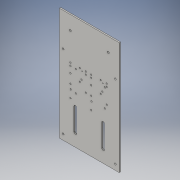
# Autodesk Inventor part: Part2
Saved by Autodesk Inventor 2016 (Build 200138000, 138)
## iProperties
Created: 2015-10-15
Part Number: Part2
Material: Generic
Document SubType Name: Modeling
Designer: hozhu
Density: 1 g/cm^3
Appearance: Default
Author: hozhu
Autodesk Inventor part; units mm, degrees
ref_plane "YZ Plane" through (0, 0, 0) normal (1, 0, 0) x (0, 1, 0)
ref_plane "XZ Plane" through (0, 0, 0) normal (0, 1, 0) x (-1, 0, 0)
ref_plane "XY Plane" through (0, 0, 0) normal (0, 0, 1) x (1, 0, 0)
sketch "Sketch1" plane through (0, 0, 0) normal (0, 0, 1) x (1, 0, 0)
  line L0 (-68.58, -128.7145) -> (68.58, -128.7145)
  line L1 (68.58, -128.7145) -> (68.58, 128.7145)
  line L2 (68.58, 128.7145) -> (-68.58, 128.7145)
  line L3 (-68.58, 128.7145) -> (-68.58, -128.7145)
  line L4 (-68.58, -128.7145) -> (68.58, 128.7145) construction
  line L5 (68.58, -128.7145) -> (-68.58, 128.7145) construction
  point P0 (0, 0)
  dimension "d0" = 137.16
  dimension "d1" = 257.429
  constraints: 12 end point, 2 midpoint, 2 parallel, 1 horizontal, 1 perpendicular
  measures "d0" distance of L1.end L2.end
  measures "d1" distance of L2.end L0.start
extrude "Extrusion1" add sketch "Sketch1" against normal blind 3.175
sketch "Sketch2" plane through (0, 0, 0) normal (0, 0, 1) x (1, 0, 0)
  circle A0 centre (-59.69, 52.5145) radius 2.0955
  line L0 (-68.58, 128.7145) -> (-68.58, -128.7145) projected
  line L1 (-68.58, 128.7145) -> (68.58, 128.7145) projected
  circle A1 centre (59.69, 52.5145) radius 2.0955
  line L2 (68.58, -128.7145) -> (68.58, 128.7145) projected
  circle A2 centre (-59.69, -116.0145) radius 2.0955
  circle A3 centre (59.69, -116.0145) radius 2.0955
  line L3 (-68.58, -128.7145) -> (68.58, -128.7145) projected
  point P0 (0, 0)
  dimension "d4" = 8.89
  dimension "d5" = 76.2
  dimension "d6" = 76.2
  dimension "d7" = 8.89
  dimension "d8" = 4.191
  dimension "d9" = 12.7
  dimension "d10" = 8.89
  dimension "d11" = 8.89
  dimension "d12" = 12.7
  dimension "d13" = 4.191
  dimension "d21" = 4.191
  dimension "d22" = 4.191
  constraints: 4 centre point
  measures "d4" distance from line of L0 A0.centre
  measures "d5" distance from line of L1 A0.centre
  measures "d6" distance from line of L1 A1.centre
  measures "d7" distance from line of A1.centre L2
  measures "d8" diameter of A1
  measures "d9" distance from line of L3 A2.centre
  measures "d10" distance from line of L0 A2.centre
  measures "d11" distance from line of L2 A3.centre
  measures "d12" distance from line of L3 A3.centre
  measures "d13" diameter of A0
  measures "d21" diameter of A2
  measures "d22" diameter of A3
hole "Hole1" at (-59.69, 52.5145, 0) at (59.69, 52.5145, 0) at (-59.69, -116.0145, 0) at (59.69, -116.0145, 0) direction (0, 0, -1) diameter 4.191 end through all
sketch "Sketch4" plane through (0, 0, 0) normal (0, 0, 1) x (1, 0, 0)
  line L0 (-35.179, -49.0855) -> (-35.179, -99.8855)
  line L1 (-28.321, -49.0855) -> (-28.321, -99.8855)
  line L2 (28.321, -49.0855) -> (28.321, -99.8855)
  line L3 (35.179, -49.0855) -> (35.179, -99.8855)
  line L4 (-68.58, 128.7145) -> (-68.58, -128.7145) projected
  line L5 (68.58, -128.7145) -> (68.58, 128.7145) projected
  line L6 (-68.58, -128.7145) -> (68.58, -128.7145) projected
  arc A0 (-28.321, -49.0855) -> (-35.179, -49.0855) centre (-31.75, -49.0855) ccw
  arc A1 (-35.179, -99.8855) -> (-28.321, -99.8855) centre (-31.75, -99.8855) ccw
  arc A2 (35.179, -49.0855) -> (28.321, -49.0855) centre (31.75, -49.0855) ccw
  arc A3 (28.321, -99.8855) -> (35.179, -99.8855) centre (31.75, -99.8855) ccw
  point P0 (0, 0)
  dimension "d23" = 6.858
  dimension "d24" = 6.858
  dimension "d25" = 33.401
  dimension "d26" = 50.8
  dimension "d27" = 33.401
  dimension "d28" = 28.829
  dimension "d29" = 28.829
  dimension "d30" = 28.829
  dimension "d31" = 28.829
  dimension "d32" = 50.8
  dimension "d33" = 50.8
  dimension "d34" = 50.8
  constraints: 8 end point, 8 point on circle, 4 centre point, 4 tangent, 4 vertical
  measures "d23" distance of L1.end L0.end
  measures "d24" distance between parallel lines of L3 L2
  measures "d25" distance between parallel lines of L4 L0
  measures "d26" distance of L3.start L3.end
  measures "d27" distance between parallel lines of L5 L3
  measures "d28" distance from line of L6 L0.end
  measures "d29" distance from line of L6 L1.end
  measures "d30" distance from line of L6 L2.end
  measures "d31" distance from line of L6 L3.end
  measures "d32" distance of L0.start L0.end
  measures "d33" distance of L1.start L1.end
  measures "d34" distance of L2.start L2.end
extrude "Extrusion2" cut sketch "Sketch4" against normal blind 3.175
sketch "Sketch5" plane through (0, 0, 0) normal (0, 0, 1) x (1, 0, 0)
  line L0 (-68.58, 128.7145) -> (68.58, 128.7145) projected
  line L1 (68.58, 128.7145) -> (68.58, -128.7145) projected
  point P0 (0, 0)
  point P1 (-43.3324, 96.9645)
  point P2 (43.3324, 96.9645)
  dimension "d37" = 31.75
  dimension "d38" = 86.6648
  dimension "d39" = 31.75
  dimension "d40" = 25.2476
  measures "d37" distance from line of L0 point (-43.332, 96.964)
  measures "d38" distance of point (-43.332, 96.964) point (43.332, 96.964)
  measures "d39" distance from line of L0 point (43.332, 96.964)
  measures "d40" distance from line of L1 point (43.332, 96.964)
hole "Hole2" at (-43.3324, 96.9645, 0) at (43.3324, 96.9645, 0) direction (0, 0, -1) diameter 4.4704 end through all
sketch "battery_buzzer" plane through (0, 0, 0) normal (0, 0, 1) x (1, 0, 0)
  line L0 (-50.8, 39.8145) -> (50.8, 39.8145)
  line L1 (50.8, 39.8145) -> (50.8, -36.3855)
  line L2 (50.8, -36.3855) -> (-50.8, -36.3855)
  line L3 (-50.8, -36.3855) -> (-50.8, 39.8145)
  line L4 (68.58, -128.7145) -> (68.58, 128.7145) projected
  line L5 (68.58, 128.7145) -> (-68.58, 128.7145) projected
  line L6 (-68.58, 128.7145) -> (-68.58, -128.7145) projected
  line L7 (-46.99, 37.2745) -> (-13.97, 37.2745)
  line L8 (-13.97, 37.2745) -> (-13.97, 9.3345)
  line L9 (-13.97, 9.3345) -> (-46.99, 9.3345)
  line L10 (-46.99, 9.3345) -> (-46.99, 37.2745)
  circle A0 centre (-43.18, 33.4645) radius 1.651
  circle A1 centre (-43.18, 12.5095) radius 1.651
  circle A2 centre (-17.78, 12.5095) radius 1.651
  line L11 (0.635, 37.2745) -> (33.655, 37.2745)
  line L12 (33.655, 37.2745) -> (33.655, 9.3345)
  line L13 (33.655, 9.3345) -> (0.635, 9.3345)
  line L14 (0.635, 9.3345) -> (0.635, 37.2745)
  circle A3 centre (4.445, 33.4645) radius 1.651
  circle A4 centre (4.445, 12.5095) radius 1.651
  circle A5 centre (29.845, 12.5095) radius 1.651
  point P0 (-1.6153, -4.4833)
  point P1 (48.3688, -4.4833)
  dimension "d48" = 17.78
  dimension "d49" = 88.9
  dimension "d50" = 76.2
  dimension "d51" = 17.78
  dimension "d52" = 33.02
  dimension "d54" = 3.302
  dimension "d55" = 3.302
  dimension "d57" = 3.81
  dimension "d58" = 3.81
  dimension "d59" = 3.81
  dimension "d60" = 20.955
  dimension "d62" = 25.4
  dimension "d74" = 33.02
  dimension "d75" = 3.302
  dimension "d76" = 3.302
  dimension "d77" = 3.81
  dimension "d78" = 3.81
  dimension "d79" = 3.81
  dimension "d80" = 20.955
  dimension "d81" = 25.4
  dimension "d190" = 25.4
  dimension "d191" = 95.25
  dimension "d192" = 73.025
  constraints: 24 end point, 7 perpendicular, 6 centre point, 3 horizontal, 2 collinear, 2 parallel
  measures "d48" distance between parallel lines of L4 L1
  measures "d49" distance between parallel lines of L5 L0
  measures "d50" distance of L0.end L1.end
  measures "d51" distance between parallel lines of L6 L3
  measures "d52" distance of L7.start L7.end
  measures "d54" diameter of A0
  measures "d55" diameter of A1
  measures "d57" distance from line of L7 A0.centre
  measures "d58" distance from line of L10 A1.centre
  measures "d59" distance from line of L10 A0.centre
  measures "d60" distance of A1.centre A0.centre
  measures "d62" distance of A1.centre A2.centre
  measures "d74" distance of L11.start L12.start
  measures "d75" diameter of A3
  measures "d76" diameter of A4
  measures "d77" distance from line of L11 A3.centre
  measures "d78" distance from line of L14 A4.centre
  measures "d79" distance from line of L14 A3.centre
  measures "d80" distance of A4.centre A3.centre
  measures "d81" distance of A4.centre A5.centre
  measures "d190" distance from line of L6 A0.centre
  measures "d191" distance from line of A0.centre L5
  measures "d192" distance from line of L6 A3.centre
sketch "grizzly_bear" plane through (0, 0, 0) normal (0, 0, 1) x (1, 0, 0)
  line L0 (-5.08, -39.9415) -> (-5.08, 36.2585)
  line L1 (-5.08, 36.2585) -> (-46.355, 36.2585)
  line L2 (-46.355, 36.2585) -> (-46.355, -39.9415)
  line L3 (-46.355, -39.9415) -> (-5.08, -39.9415)
  circle A0 centre (-43.18, -36.8935) radius 1.651
  circle A1 centre (-7.874, 33.4645) radius 1.651
  circle A2 centre (-43.18, 33.4645) radius 1.651
  line L4 (42.545, -39.9415) -> (42.545, 36.2585)
  line L5 (42.545, 36.2585) -> (1.27, 36.2585)
  line L6 (1.27, 36.2585) -> (1.27, -39.9415)
  line L7 (1.27, -39.9415) -> (42.545, -39.9415)
  circle A3 centre (4.445, -36.8935) radius 1.651
  circle A4 centre (39.751, 33.4645) radius 1.651
  circle A5 centre (4.445, 33.4645) radius 1.651
  line L8 (-68.58, 128.7145) -> (-68.58, -128.7145) projected
  line L9 (68.58, 128.7145) -> (-68.58, 128.7145) projected
  point P0 (0, 0)
  point P1 (53.9394, 0)
  dimension "d83" = 3.302
  dimension "d85" = 76.2
  dimension "d86" = 41.275
  dimension "d89" = 2.794
  dimension "d90" = 3.175
  dimension "d91" = 2.794
  dimension "d92" = 38.481
  dimension "d97" = 73.152
  dimension "d98" = 3.175
  dimension "d166" = 3.302
  dimension "d168" = 76.2
  dimension "d169" = 41.275
  dimension "d172" = 2.794
  dimension "d173" = 3.175
  dimension "d174" = 2.794
  dimension "d175" = 38.481
  dimension "d180" = 73.152
  dimension "d181" = 3.175
  dimension "d182" = 6.35
  dimension "d188" = 95.25
  dimension "d189" = 25.4
  constraints: 16 end point, 6 centre point, 5 parallel, 4 equal radius, 1 collinear, 1 horizontal, 1 perpendicular
  measures "d83" diameter of A2
  measures "d85" distance between parallel lines of L1 L3
  measures "d86" distance between parallel lines of L2 L0
  measures "d89" distance from line of A2.centre L1
  measures "d90" distance from line of A2.centre L2
  measures "d91" distance from line of A1.centre L1
  measures "d92" distance from line of A1.centre L2
  measures "d97" distance from line of A0.centre L1
  measures "d98" distance from line of A0.centre L2
  measures "d166" diameter of A5
  measures "d168" distance between parallel lines of L5 L7
  measures "d169" distance between parallel lines of L6 L4
  measures "d172" distance from line of A5.centre L5
  measures "d173" distance from line of A5.centre L6
  measures "d174" distance from line of A4.centre L5
  measures "d175" distance from line of A4.centre L6
  measures "d180" distance from line of A3.centre L5
  measures "d181" distance from line of A3.centre L6
  measures "d182" distance of L5.end L0.end
  measures "d188" distance from line of L9 A2.centre
  measures "d189" distance from line of L8 A2.centre
sketch "Smartsensor" plane through (0, 0, 0) normal (0, 0, 1) x (1, 0, 0)
  line L0 (-46.99, 9.3345) -> (-46.99, 37.2745)
  line L1 (-46.99, 37.2745) -> (-13.97, 37.2745)
  line L2 (-13.97, 37.2745) -> (-13.97, 9.3345)
  line L3 (-46.99, 9.3345) -> (-13.97, 9.3345)
  circle A0 centre (-43.18, 33.4645) radius 1.651
  circle A1 centre (-17.78, 12.5095) radius 1.651
  circle A2 centre (-16.51, 29.6545) radius 1
  line L4 (0.635, 9.3345) -> (0.635, 37.2745)
  line L5 (0.635, 37.2745) -> (33.655, 37.2745)
  line L6 (33.655, 37.2745) -> (33.655, 9.3345)
  line L7 (0.635, 9.3345) -> (33.655, 9.3345)
  circle A3 centre (4.445, 33.4645) radius 1.651
  circle A4 centre (29.845, 12.5095) radius 1.651
  circle A5 centre (31.115, 29.6545) radius 1
  point P0 (0, 0)
  point P1 (4.445, 33.4645)
  constraints: 16 end point, 6 centre point, 2 collinear
sketch "SmartsensorPowered" plane through (0, 0, 0) normal (0, 0, 1) x (1, 0, 0)
  line L0 (-46.355, 36.6395) -> (-18.415, 36.6395)
  line L1 (-18.415, 36.6395) -> (-18.415, -23.0505)
  line L2 (-18.415, -23.0505) -> (-46.355, -23.0505)
  line L3 (-46.355, -23.0505) -> (-46.355, 36.6395)
  circle A0 centre (-43.18, 33.4645) radius 1.651
  circle A1 centre (-21.59, 33.4645) radius 1.651
  circle A2 centre (-42.545, -19.2405) radius 1.651
  circle A3 centre (-21.59, 6.1595) radius 1.651
  line L4 (-68.58, 128.7145) -> (-68.58, -128.7145) projected
  line L5 (68.58, 128.7145) -> (-68.58, 128.7145) projected
  line L6 (1.27, 36.6395) -> (29.21, 36.6395)
  line L7 (29.21, 36.6395) -> (29.21, -23.0505)
  line L8 (29.21, -23.0505) -> (1.27, -23.0505)
  line L9 (1.27, -23.0505) -> (1.27, 36.6395)
  circle A4 centre (4.445, 33.4645) radius 1.651
  circle A5 centre (26.035, 33.4645) radius 1.651
  circle A6 centre (5.08, -19.2405) radius 1.651
  circle A7 centre (26.035, 6.1595) radius 1.651
  dimension "d99" = 59.69
  dimension "d100" = 27.94
  dimension "d101" = 3.302
  dimension "d102" = 3.302
  dimension "d103" = 3.302
  dimension "d104" = 3.302
  dimension "d105" = 3.175
  dimension "d106" = 3.81
  dimension "d107" = 3.175
  dimension "d108" = 3.81
  dimension "d109" = 3.175
  dimension "d110" = 3.175
  dimension "d111" = 3.175
  dimension "d112" = 30.48
  dimension "d186" = 25.4
  dimension "d187" = 95.25
  dimension "d193" = 59.69
  dimension "d194" = 27.94
  dimension "d195" = 3.302
  dimension "d196" = 3.302
  dimension "d197" = 3.302
  dimension "d198" = 3.302
  dimension "d199" = 3.175
  dimension "d200" = 3.81
  dimension "d201" = 3.175
  dimension "d202" = 3.81
  dimension "d203" = 3.175
  dimension "d204" = 3.175
  dimension "d205" = 3.175
  dimension "d206" = 30.48
  dimension "d207" = 73.025
  constraints: 16 end point, 8 centre point, 4 parallel, 2 horizontal, 2 perpendicular
  measures "d99" distance of L2.end L0.start
  measures "d100" distance of L0.start L0.end
  measures "d101" diameter of A0
  measures "d102" diameter of A1
  measures "d103" diameter of A3
  measures "d104" diameter of A2
  measures "d105" distance from line of L3 A0.centre
  measures "d106" distance from line of L3 A2.centre
  measures "d107" distance from line of A0.centre L0
  measures "d108" distance from line of L2 A2.centre
  measures "d109" distance from line of L1 A1.centre
  measures "d110" distance from line of L1 A3.centre
  measures "d111" distance from line of A1.centre L0
  measures "d112" distance from line of L0 A3.centre
  measures "d186" distance from line of L4 A0.centre
  measures "d187" distance from line of L5 A0.centre
  measures "d193" distance of L8.end L6.start
  measures "d194" distance of L6.start L7.start
  measures "d195" diameter of A4
  measures "d196" diameter of A5
  measures "d197" diameter of A7
  measures "d198" diameter of A6
  measures "d199" distance from line of L9 A4.centre
  measures "d200" distance from line of L9 A6.centre
  measures "d201" distance from line of A4.centre L6
  measures "d202" distance from line of L8 A6.centre
  measures "d203" distance from line of L7 A5.centre
  measures "d204" distance from line of L7 A7.centre
  measures "d205" distance from line of A5.centre L6
  measures "d206" distance from line of L6 A7.centre
  measures "d207" distance from line of L4 A4.centre
sketch "teamflag" plane through (0, 0, 0) normal (0, 0, 1) x (1, 0, 0)
  line L0 (-45.72, 29.6545) -> (-5.08, 29.6545)
  line L1 (-5.08, 29.6545) -> (-5.08, -10.9855)
  line L2 (-5.08, -10.9855) -> (-45.72, -10.9855)
  line L3 (-45.72, -10.9855) -> (-45.72, 29.6545)
  circle A0 centre (-43.18, 27.1145) radius 1.651
  circle A1 centre (-43.18, -8.4455) radius 1.651
  circle A2 centre (-7.62, 27.1145) radius 1.651
  circle A3 centre (-7.62, -8.4455) radius 1.651
  line L4 (1.905, 29.6545) -> (42.545, 29.6545)
  line L5 (42.545, 29.6545) -> (42.545, -10.9855)
  line L6 (42.545, -10.9855) -> (1.905, -10.9855)
  line L7 (1.905, -10.9855) -> (1.905, 29.6545)
  circle A4 centre (4.445, 27.1145) radius 1.651
  circle A5 centre (4.445, -8.4455) radius 1.651
  circle A6 centre (40.005, 27.1145) radius 1.651
  circle A7 centre (40.005, -8.4455) radius 1.651
  line L8 (-68.58, 128.7145) -> (-68.58, -128.7145) projected
  line L9 (68.58, 128.7145) -> (-68.58, 128.7145) projected
  point P0 (0, 0)
  point P1 (-43.18, 33.4645)
  point P2 (4.445, 33.4645)
  point P3 (-42.545, -19.2405)
  point P4 (5.08, -19.2405)
  point P5 (-43.18, 33.4645)
  point P6 (4.445, 27.1145)
  dimension "d128" = 40.64
  dimension "d129" = 40.64
  dimension "d140" = 35.56
  dimension "d141" = 35.56
  dimension "d142" = 35.56
  dimension "d143" = 2.54
  dimension "d144" = 2.54
  dimension "d145" = 40.64
  dimension "d146" = 40.64
  dimension "d147" = 35.56
  dimension "d148" = 35.56
  dimension "d149" = 35.56
  dimension "d150" = 2.54
  dimension "d151" = 2.54
  dimension "d209" = 25.4
  dimension "d210" = 101.6
  dimension "d211" = 73.025
  dimension "d212" = 101.6
  constraints: 16 end point, 8 centre point, 6 equal radius, 4 parallel, 2 horizontal, 2 perpendicular
  measures "d128" distance of L0.start L0.end
  measures "d129" distance of L2.end L0.start
  measures "d140" distance of A2.centre A0.centre
  measures "d141" distance of A0.centre A1.centre
  measures "d142" distance of A3.centre A1.centre
  measures "d143" distance from line of L1 A2.centre
  measures "d144" distance from line of L0 A2.centre
  measures "d145" distance of L4.start L4.end
  measures "d146" distance of L6.end L4.start
  measures "d147" distance of A6.centre A4.centre
  measures "d148" distance of A4.centre A5.centre
  measures "d149" distance of A7.centre A5.centre
  measures "d150" distance from line of L5 A6.centre
  measures "d151" distance from line of L4 A6.centre
  measures "d209" distance from line of L8 point (-43.18, 27.114)
  measures "d210" distance from line of L9 point (-43.18, 27.114)
  measures "d211" distance from line of L8 point (4.445, 27.114)
  measures "d212" distance from line of L9 point (4.445, 27.114)
sketch "cape" plane through (0, 0, 0) normal (0, 0, 1) x (1, 0, 0)
  line L0 (-33.655, 30.2793) -> (38.4048, 30.2793)
  line L1 (38.4048, 30.2793) -> (38.4048, -24.3205)
  line L2 (38.4048, -24.3205) -> (-33.655, -24.3205)
  line L3 (-33.655, -24.3205) -> (-33.655, 30.2793)
  circle A0 centre (-30.48, 27.1145) radius 1.5875
  circle A1 centre (-30.48, -21.1455) radius 1.5875
  circle A2 centre (35.56, 23.9395) radius 1.5875
  circle A3 centre (35.56, -17.9705) radius 1.5875
  line L4 (-68.58, 128.7145) -> (-68.58, -128.7145) projected
  point P0 (0, 0)
  point P1 (-43.18, 33.4645)
  point P2 (-43.18, 27.1145)
  point P3 (-42.545, -19.2405)
  point P4 (-30.48, 27.1145)
  point P5 (-24.13, 20.7645)
  dimension "d152" = 3.175
  dimension "d153" = 72.0598
  dimension "d154" = 54.5998
  dimension "d155" = 48.26
  dimension "d156" = 0
  dimension "d157" = 3.175
  dimension "d158" = 3.175
  dimension "d159" = 41.91
  dimension "d160" = 0
  dimension "d161" = 6.35
  dimension "d162" = 2.8448
  dimension "d269" = 38.1
  dimension "d270" = 44.45
  constraints: 8 end point, 4 centre point, 3 equal radius, 2 parallel, 1 horizontal, 1 perpendicular
  measures "d152" diameter of A0
  measures "d153" distance of L0.start L0.end
  measures "d154" distance of L2.end L0.start
  measures "d155" distance of A1.centre A0.centre
  measures "d156" horizontal distance of A1.centre A0.centre
  measures "d157" distance from line of L3 A0.centre
  measures "d158" distance from line of L2 A1.centre
  measures "d159" distance of A3.centre A2.centre
  measures "d160" horizontal distance of A3.centre A2.centre
  measures "d161" distance from line of L2 A3.centre
  measures "d162" distance from line of L1 A2.centre
  measures "d269" distance from line of L4 point (-30.48, 27.114)
  measures "d270" distance from line of L4 point (-24.13, 20.764)
sketch "Board Area" plane through (0, 0, 0) normal (0, 0, 1) x (1, 0, 0)
  line L0 (-50.8, 39.8145) -> (50.8, 39.8145)
  line L1 (50.8, 39.8145) -> (50.8, -128.7145)
  line L2 (50.8, -128.7145) -> (-50.8, -128.7145)
  line L3 (-50.8, -128.7145) -> (-50.8, 39.8145)
  line L4 (68.58, 128.7145) -> (-68.58, 128.7145) projected
  line L5 (-68.58, 128.7145) -> (-68.58, -128.7145) projected
  line L6 (-68.58, -128.7145) -> (68.58, -128.7145) projected
  point P0 (0, 0)
  dimension "d163" = 101.6
  dimension "d164" = 88.9
  dimension "d165" = 17.78
  constraints: 8 end point, 2 parallel, 1 collinear, 1 horizontal, 1 perpendicular
  measures "d163" distance between parallel lines of L1 L3
  measures "d164" distance between parallel lines of L0 L4
  measures "d165" distance between parallel lines of L5 L3
hole "Hole3" at (-43.18, 27.1145, 0) at (-43.18, -8.4455, 0) at (-7.62, -8.4455, 0) at (-7.62, 27.1145, 0) at (4.445, 27.1145, 0) at (4.445, -8.4455, 0) at (40.005, -8.4455, 0) at (40.005, 27.1145, 0) direction (0, 0, -1) diameter 3.302 end through all
hole "Hole5" at (-43.18, -36.8935, 0) at (4.445, -36.8935, 0) at (39.751, 33.4645, 0) at (-7.874, 33.4645, 0) direction (0, 0, -1) diameter 3.302 end through all
hole "Hole6" at (-17.78, 12.5095, 0) at (29.845, 12.5095, 0) direction (0, 0, -1) diameter 3.302 end through all
hole "Hole7" at (-43.18, 12.5095, 0) at (4.445, 12.5095, 0) direction (0, 0, -1) diameter 3.302 end through all
hole "Hole9" at (-43.18, 33.4645, 0) at (4.445, 33.4645, 0) at (-16.51, 29.6545, 0) direction (0, 0, -1) diameter 2.0066 end through all
hole "Hole10" at (31.115, 29.6545, 0) direction (0, 0, -1) diameter 2.0066 end through all
hole "Hole11" at (-30.48, 27.1145, 0) at (-30.48, -21.1455, 0) at (35.56, -17.9705, 0) at (35.56, 23.9395, 0) direction (0, 0, -1) diameter 3.302 end through all
hole "Hole12" at (-42.545, -19.2405, 0) at (-21.59, 33.4645, 0) at (26.035, 33.4645, 0) at (5.08, -19.2405, 0) at (4.445, 33.4645, 0) at (-43.18, 33.4645, 0) at (-21.59, 6.1595, 0) at (26.035, 6.1595, 0) direction (0, 0, -1) diameter 3.302 end through all
body "Solid1"
